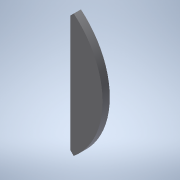
# Autodesk Inventor part: Tapa baterías
Saved by Autodesk Inventor 2021.3 (Build 253353010, 353A)
## iProperties
Created: 2021-09-07
Part Number: Tapa baterías
Material: Generic
Document SubType Name: Modeling
Designer: pili2
Density: 1 g/cm^3
Appearance: Default
Author: pili2
Autodesk Inventor part; units mm, degrees
ref_plane "YZ Plane" through (0, 0, 0) normal (1, 0, 0) x (0, 1, 0)
ref_plane "XZ Plane" through (0, 0, 0) normal (0, 1, 0) x (-1, 0, 0)
ref_plane "XY Plane" through (0, 0, 0) normal (0, 0, 1) x (1, 0, 0)
sketch "Sketch1" plane through (0, 0, 0) normal (0, 0, 1) x (1, 0, 0)
  line L0 (2.9368, 14.113) -> (2.9368, -34.387)
  line L1 (2.9368, 14.113) -> (4.3998, 15.576)
  line L2 (2.9368, 14.113) -> (5.0058, 14.113) construction
  line L3 (2.9368, -34.387) -> (4.3998, -35.85)
  line L4 (2.9368, -34.387) -> (5.0058, -34.387) construction
  arc A0 (4.3998, -35.85) -> (4.3998, 15.576) centre (-17.0632, -10.137) ccw
  point P0 (0, 0)
  point P1 (2.9368, -10.137)
  dimension "d0" = 48.5
  dimension "d1" = 2.069
  dimension "d2" = 45
  dimension "d3" = 2.069
  dimension "d4" = 45
  dimension "d7" = 20
  constraints: 11 end point, 2 equal length, 2 horizontal, 2 point on circle, 2 vertical, 1 centre point, 1 horizontal alignment, 1 midpoint, 1 point on line
  measures "d0" distance of L0.start L0.end
  measures "d1" distance of L1.end L0.start
  measures "d2" angle of L2 L1
  measures "d3" distance of L0.end L3.end
  measures "d4" angle of L3 L4
  measures "d7" distance from line of L0 A0.centre
extrude "Extrusion1" add sketch "Sketch1" against normal blind 3
body "Solid1"
